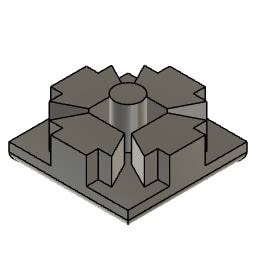
LDO_2020_Cap (Autodesk Fusion 360 design; units mm, degrees)
Autodesk Fusion 360 part; units mm, degrees
sketch "Base" plane through (0, 0, 0) normal (0, 0, 1) x (1, 0, 0)
  line L0 (10, -10) -> (-10, -10)
  line L1 (-10, -10) -> (-10, 10)
  line L2 (-10, 10) -> (10, 10)
  line L3 (10, 10) -> (10, -10)
  line L4 (10, -10) -> (-10, 10) construction
  line L5 (-10, -10) -> (10, 10) construction
  circle A0 centre (0, 0) radius 2.25
  dimension "d1" = 20
  dimension "d2" = 20
  dimension "d3" = 4.5
  constraint horizontal L0
  constraint perpendicular L0 L1
  constraint parallel L0 L2
  constraint parallel L1 L3
  constraint coincident L4 A0.centre
  constraint coincident L5 A0.centre
  constraint coincident A0.centre origin
  measures "d1" distance of L1.end L2.end
  measures "d2" distance of L0.end L1.end
  measures "d3" diameter of A0
extrude "Extrude1" add sketch "Base" along normal blind 3
extrude "Extrude2" add sketch "Base" along normal blind 10 contours A0
fillet "Fillet1" radius 1.5 4 edges at (10, 0, 0) (0, 10, 0) (-10, 0, 0) (0, -10, 0)
sketch "Inserts" plane through (0, 0, 0) normal (0, 0, 1) x (1, 0, 0)
  line L0 (-10, -10) -> (-3, -10)
  line L1 (-3, -10) -> (3, -10)
  line L2 (3, -10) -> (3, -8)
  line L3 (-3, -10) -> (-3, -8)
  line L4 (-3, -8) -> (-3, -3.6)
  line L5 (-3, -3.6) -> (3, -3.6)
  line L6 (3, -8) -> (5.25, -8)
  line L7 (-3, -8) -> (-5.25, -8)
  line L8 (-5.25, -8) -> (-3, -3.6)
  line L9 (5.25, -8) -> (3, -3.6)
  line L10 (-3, -8) -> (3, -8)
  line L11 (-10, 3) -> (-10, -3)
  line L12 (-8, 3) -> (-3.6, 3)
  line L13 (-8, -3) -> (-8, -5.25)
  line L14 (-3.6, 3) -> (-3.6, -3)
  line L15 (-8, 3) -> (-8, -3)
  line L16 (-8, 5.25) -> (-3.6, 3)
  line L17 (-10, 10) -> (-10, 3)
  line L18 (-8, 3) -> (-8, 5.25)
  line L19 (-8, -5.25) -> (-3.6, -3)
  line L20 (-10, 3) -> (-8, 3)
  line L21 (-10, -3) -> (-8, -3)
  line L22 (3, 10) -> (-3, 10)
  line L23 (3, 8) -> (3, 3.6)
  line L24 (-3, 8) -> (-5.25, 8)
  line L25 (3, 3.6) -> (-3, 3.6)
  line L26 (3, 8) -> (-3, 8)
  line L27 (5.25, 8) -> (3, 3.6)
  line L28 (10, 10) -> (3, 10)
  line L29 (3, 8) -> (5.25, 8)
  line L30 (-5.25, 8) -> (-3, 3.6)
  line L31 (3, 10) -> (3, 8)
  line L32 (-3, 10) -> (-3, 8)
  line L33 (10, -3) -> (10, 3)
  line L34 (8, -3) -> (3.6, -3)
  line L35 (8, 3) -> (8, 5.25)
  line L36 (3.6, -3) -> (3.6, 3)
  line L37 (8, -3) -> (8, 3)
  line L38 (8, -5.25) -> (3.6, -3)
  line L39 (10, -10) -> (10, -3)
  line L40 (8, -3) -> (8, -5.25)
  line L41 (8, 5.25) -> (3.6, 3)
  line L42 (10, -3) -> (8, -3)
  line L43 (10, 3) -> (8, 3)
  point P0 (-10, -10)
  point P1 (-10, 10)
  point P2 (10, 10)
  point P3 (10, -10)
  dimension "d10" = 7
  dimension "d11" = 6
  dimension "d12" = 2
  dimension "d13" = 2
  dimension "d14" = 4.4
  dimension "d15" = 6
  dimension "d16" = 2.25
  dimension "d17" = 2.25
  dimension "d27" = 7
  dimension "d28" = 6
  dimension "d29" = 2
  dimension "d30" = 2
  dimension "d31" = 4.4
  dimension "d32" = 6
  dimension "d33" = 2.25
  dimension "d34" = 2.25
  dimension "d35" = 7
  dimension "d36" = 6
  dimension "d37" = 2
  dimension "d38" = 2
  dimension "d39" = 4.4
  dimension "d40" = 6
  dimension "d41" = 2.25
  dimension "d42" = 2.25
  dimension "d43" = 7
  dimension "d44" = 6
  dimension "d45" = 2
  dimension "d46" = 2
  dimension "d47" = 4.4
  dimension "d48" = 6
  dimension "d49" = 2.25
  dimension "d50" = 2.25
  constraint coincident P0 L0.start
  constraint parallel L0 L1
  constraint perpendicular L1 L2
  constraint perpendicular L1 L3
  constraint parallel L3 L4
  constraint perpendicular L4 L5
  constraint perpendicular L2 L6
  constraint perpendicular L3 L7
  constraint coincident P1 L17.start
  constraint parallel L11 L17
  constraint perpendicular L11 L21
  constraint perpendicular L11 L20
  constraint parallel L12 L20
  constraint perpendicular L12 L14
  constraint perpendicular L13 L21
  constraint perpendicular L18 L20
  constraint coincident P2 L28.start
  constraint parallel L22 L28
  constraint perpendicular L22 L32
  constraint perpendicular L22 L31
  constraint parallel L23 L31
  constraint perpendicular L23 L25
  constraint perpendicular L24 L32
  constraint perpendicular L29 L31
  constraint coincident P3 L39.start
  constraint parallel L33 L39
  constraint perpendicular L33 L43
  constraint perpendicular L33 L42
  constraint parallel L34 L42
  constraint perpendicular L34 L36
  constraint perpendicular L35 L43
  constraint perpendicular L40 L42
  measures "d10" distance of P0 L0.end
  measures "d11" distance of L0.end L1.end
  measures "d12" distance of L1.end L2.end
  measures "d13" distance of L0.end L3.end
  measures "d14" distance of L3.end L4.end
  measures "d15" distance of L4.end L5.end
  measures "d16" distance of L2.end L6.end
  measures "d17" distance of L3.end L7.end
  measures "d27" distance of P1 L11.start
  measures "d28" distance of L11.end L11.start
  measures "d29" distance of L11.end L13.start
  measures "d30" distance of L11.start L12.start
  measures "d31" distance of L12.end L12.start
  measures "d32" distance of L12.end L14.end
  measures "d33" distance of L13.start L13.end
  measures "d34" distance of L16.start L12.start
  measures "d35" distance of P2 L22.start
  measures "d36" distance of L22.end L22.start
  measures "d37" distance of L22.end L24.start
  measures "d38" distance of L22.start L23.start
  measures "d39" distance of L23.end L23.start
  measures "d40" distance of L23.end L25.end
  measures "d41" distance of L24.start L24.end
  measures "d42" distance of L27.start L23.start
  measures "d43" distance of P3 L33.start
  measures "d44" distance of L33.end L33.start
  measures "d45" distance of L33.end L35.start
  measures "d46" distance of L33.start L34.start
  measures "d47" distance of L34.end L34.start
  measures "d48" distance of L34.end L36.end
  measures "d49" distance of L35.start L35.end
  measures "d50" distance of L38.start L34.start
extrude "Extrude4" add sketch "Inserts" along normal blind 3 from surface at 3 contours L1 L2 L3 L10 | L4 L7 L8 | L4 L5 L6 L9 L10
extrude "Extrude5" add sketch "Inserts" along normal blind 4.5 from surface at 3 contours L1 L2 L3 L10 | L4 L7 L8 | L4 L5 L6 L9 L10
extrude "Extrude6" add sketch "Inserts" along normal blind 3 from surface at 3 contours L11 L15 L20 L21 | L12 L16 L18 | L12 L13 L14 L15 L19 | L22 L26 L31 L32 | L23 L27 L29 | L23 L24 L25 L26 L30 | L33 L37 L42 L43 | L34 L38 L40 | L34 L35 L36 L37 L41
extrude "Extrude7" add sketch "Inserts" along normal blind 4.5 from surface at 3 contours L11 L15 L20 L21 | L12 L16 L18 | L12 L13 L14 L15 L19 | L22 L26 L31 L32 | L23 L27 L29 | L23 L24 L25 L26 L30 | L33 L37 L42 L43 | L34 L38 L40 | L34 L35 L36 L37 L41
named bodies: "2020_Cap"
